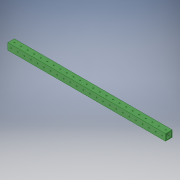
# Autodesk Inventor part: kermit frame 7
Saved by Autodesk Inventor 2018.2 (Build 222227000, 227)
## iProperties
Created: 2018-02-03
Part Number: kermit frame 7
Material: Generic
Document SubType Name: Modeling
Designer: cruz.anthony
Density: 1 g/cm^3
Appearance: Smooth - Dark Forest Green
Author: cruz.anthony
Autodesk Inventor part; units mm, degrees
ref_plane "YZ Plane" through (0, 0, 0) normal (1, 0, 0) x (0, 1, 0)
ref_plane "XZ Plane" through (0, 0, 0) normal (0, 1, 0) x (-1, 0, 0)
ref_plane "XY Plane" through (0, 0, 0) normal (0, 0, 1) x (1, 0, 0)
sketch "Sketch1" plane through (0, 0, 0) normal (0, 1, 0) x (-1, 0, 0)
  line L0 (0, 0) -> (609.6, 0)
  line L1 (609.6, 0) -> (609.6, -25.4)
  line L2 (609.6, -25.4) -> (0, -25.4)
  line L3 (0, -25.4) -> (0, 0)
  dimension "d0" = 609.6
  dimension "d1" = 25.4
  constraints: 8 end point, 2 parallel, 1 horizontal, 1 perpendicular
  measures "d0" distance of L1.end L2.end
  measures "d1" distance of L0.end L1.end
extrude "Extrusion1" add sketch "Sketch1" along normal blind 25.4
sketch "Sketch2" plane through (0, 0, 0) normal (1, 0, 0) x (0, 0, -1)
  line L0 (3.175, 22.225) -> (22.225, 22.225)
  line L1 (22.225, 22.225) -> (22.225, 3.175)
  line L2 (22.225, 3.175) -> (3.175, 3.175)
  line L3 (3.175, 3.175) -> (3.175, 22.225)
  line L4 (0, 25.4) -> (25.4, 25.4) projected
  line L5 (0, 0) -> (0, 25.4) projected
  line L6 (25.4, 0) -> (0, 0) projected
  line L7 (25.4, 0) -> (25.4, 25.4) projected
  dimension "d4" = 3.175
  dimension "d5" = 3.175
  dimension "d6" = 3.175
  dimension "d7" = 3.175
  constraints: 8 end point, 2 parallel, 1 horizontal, 1 perpendicular
  measures "d4" distance between parallel lines of L4 L0
  measures "d5" distance between parallel lines of L5 L3
  measures "d6" distance between parallel lines of L6 L2
  measures "d7" distance between parallel lines of L7 L1
extrude "Extrusion2" cut sketch "Sketch2" against normal blind 609.6 contours L0 L1 L2 L3
sketch "Sketch3" plane through (0, 0, -25.4) normal (0, 0, -1) x (-1, 0, 0)
  circle A0 centre (12.7, 12.7) radius 1.9685
  line L0 (0, 25.4) -> (609.6, 25.4) projected
  line L1 (0, 0) -> (0, 25.4) projected
  circle A1 centre (38.1, 12.7) radius 1.9685
  circle A2 centre (63.5, 12.7) radius 1.9685
  circle A3 centre (88.9, 12.7) radius 1.9685
  circle A4 centre (114.3, 12.7) radius 1.9685
  circle A5 centre (139.7, 12.7) radius 1.9685
  circle A6 centre (165.1, 12.7) radius 1.9685
  circle A7 centre (190.5, 12.7) radius 1.9685
  circle A8 centre (215.9, 12.7) radius 1.9685
  circle A9 centre (241.3, 12.7) radius 1.9685
  circle A10 centre (266.7, 12.7) radius 1.9685
  circle A11 centre (292.1, 12.7) radius 1.9685
  circle A12 centre (317.5, 12.7) radius 1.9685
  circle A13 centre (342.9, 12.7) radius 1.9685
  circle A14 centre (368.3, 12.7) radius 1.9685
  circle A15 centre (393.7, 12.7) radius 1.9685
  circle A16 centre (419.1, 12.7) radius 1.9685
  circle A17 centre (444.5, 12.7) radius 1.9685
  circle A18 centre (469.9, 12.7) radius 1.9685
  circle A19 centre (495.3, 12.7) radius 1.9685
  circle A20 centre (520.7, 12.7) radius 1.9685
  circle A21 centre (546.1, 12.7) radius 1.9685
  circle A22 centre (571.5, 12.7) radius 1.9685
  circle A23 centre (596.9, 12.7) radius 1.9685
  dimension "d10" = 3.937
  dimension "d11" = 12.7
  dimension "d12" = 12.7
  dimension "d15" = 25.4
  constraints: 24 centre point, 1 horizontal, 46 other
  measures "d10" diameter of A0
  measures "d11" distance from line of L0 A0.centre
  measures "d12" distance from line of L1 A0.centre
  measures "d15" distance of A0.centre A1.centre
extrude "Extrusion3" cut sketch "Sketch3" against normal blind 25.4
sketch "Sketch4" plane through (0, 25.4, 0) normal (0, 1, 0) x (1, 0, 0)
  circle A0 centre (-12.7, 12.7) radius 1.9685
  line L0 (-609.6, 0) -> (0, 0) projected
  line L1 (0, 0) -> (0, 25.4) projected
  circle A1 centre (-38.1, 12.7) radius 1.9685
  circle A2 centre (-63.5, 12.7) radius 1.9685
  circle A3 centre (-88.9, 12.7) radius 1.9685
  circle A4 centre (-114.3, 12.7) radius 1.9685
  circle A5 centre (-139.7, 12.7) radius 1.9685
  circle A6 centre (-165.1, 12.7) radius 1.9685
  circle A7 centre (-190.5, 12.7) radius 1.9685
  circle A8 centre (-215.9, 12.7) radius 1.9685
  circle A9 centre (-241.3, 12.7) radius 1.9685
  circle A10 centre (-266.7, 12.7) radius 1.9685
  circle A11 centre (-292.1, 12.7) radius 1.9685
  circle A12 centre (-317.5, 12.7) radius 1.9685
  circle A13 centre (-342.9, 12.7) radius 1.9685
  circle A14 centre (-368.3, 12.7) radius 1.9685
  circle A15 centre (-393.7, 12.7) radius 1.9685
  circle A16 centre (-419.1, 12.7) radius 1.9685
  circle A17 centre (-444.5, 12.7) radius 1.9685
  circle A18 centre (-469.9, 12.7) radius 1.9685
  circle A19 centre (-495.3, 12.7) radius 1.9685
  circle A20 centre (-520.7, 12.7) radius 1.9685
  circle A21 centre (-546.1, 12.7) radius 1.9685
  circle A22 centre (-571.5, 12.7) radius 1.9685
  circle A23 centre (-596.9, 12.7) radius 1.9685
  dimension "d22" = 3.937
  dimension "d23" = 12.7
  dimension "d24" = 12.7
  dimension "d27" = 25.4
  constraints: 24 centre point, 1 horizontal, 46 other
  measures "d22" diameter of A0
  measures "d23" distance from line of L0 A0.centre
  measures "d24" distance from line of L1 A0.centre
  measures "d27" distance of A0.centre A1.centre
extrude "Extrusion4" cut sketch "Sketch4" against normal blind 25.4
body "Solid1"
